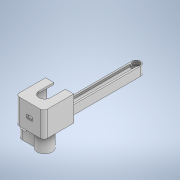
# Autodesk Inventor part: motor-rack
Saved by Autodesk Inventor 2021 (Build 250183000, 183)
## iProperties
Created: 2024-04-10
Part Number: motor-rack
Material: Generic
Document SubType Name: Modeling
Designer: 22hamfri
Density: 1 g/cm^3
Appearance: Default
Author: 22hamfri
Autodesk Inventor part; units mm, degrees
ref_plane "YZ Plane" through (0, 0, 0) normal (1, 0, 0) x (0, 1, 0)
ref_plane "XZ Plane" through (0, 0, 0) normal (0, 1, 0) x (-1, 0, 0)
ref_plane "XY Plane" through (0, 0, 0) normal (0, 0, 1) x (1, 0, 0)
sketch "Sketch1" plane through (0, 0, 0) normal (0, 1, 0) x (-1, 0, 0)
  circle A0 centre (0, -95.64) radius 2.575
  circle A1 centre (0, -95.64) radius 3.1
  circle A2 centre (0, -95.64) radius 3.8
  circle A3 centre (-15.94, 0) radius 2.575
  circle A4 centre (-15.94, 0) radius 3.1
  circle A5 centre (-15.94, 0) radius 3.8
  circle A6 centre (0, 0) radius 3.8
  line L0 (0, 0) -> (0, -95.64)
  line L1 (0, 0) -> (-15.94, 0)
  line L2 (3.8, 0) -> (3.8, -95.64)
  line L3 (-3.8, 0) -> (-3.8, -95.64)
  line L4 (0, 3.8) -> (-15.94, 3.8)
  line L5 (0, -3.8) -> (-15.94, -3.8)
  arc A7 (-3.8, -4.8) -> (-4.8, -3.8) centre (-4.8, -4.8) ccw
  line L6 (-12.9151, 2.3) -> (0, 2.3)
  line L7 (2.3, 0) -> (2.3, -92.6151)
  circle A8 centre (0, 0) radius 2.3
  arc A9 (-2.3, -4.8) -> (-4.8, -2.3) centre (-4.8, -4.8) ccw
  line L8 (-4.8, -2.3) -> (-12.9151, -2.3)
  line L9 (-2.3, -4.8) -> (-2.3, -92.6151)
  dimension "d0" = 0.7
  dimension "d1" = 6.2
  dimension "d2" = 5.15
  dimension "d3" = 0.7
  dimension "d4" = 5.15
  dimension "d5" = 6.2
  dimension "d6" = 7.6
  dimension "d7" = 95.64
  dimension "d8" = 15.94
  dimension "d9" = 1
  dimension "d10" = 1.5
  dimension "d11" = 1.5
  constraints: 20 end point, 18 point on circle, 12 tangent, 10 centre point, 4 point on line, 3 horizontal, 2 vertical, 1 coincident, 1 parallel
  measures "d0" radial gap between concentric circles of A1 A2
  measures "d1" diameter of A1
  measures "d2" diameter of A0
  measures "d3" radial gap between concentric circles of A4 A5
  measures "d4" diameter of A3
  measures "d5" diameter of A4
  measures "d6" diameter of A6
  measures "d7" distance of L0.start L0.end
  measures "d8" distance of L0.start L1.end
  measures "d9" radius of A7
  measures "d10" radial gap between concentric circles of A6 A8
  measures "d11" radial gap between concentric circles of A7 A9
extrude "Extrusion1" add sketch "Sketch1" against normal mid plane 7.76 contours A2 | A2 L7 A6 L2 | L3 L5 A9 L9 A2 | A6 L7 A8 L6 | A7 L5 L3 | A6 L6 A5 L4 | L5 A5 L8 A9 L3 | L3 A9 L5 | A5
extrude "Extrusion2" add sketch "Sketch1" against normal mid plane 6.16 contours A1 | A4
extrude "Extrusion3" add sketch "Sketch1" against normal mid plane 4 contours A2 L0 A6 L7 | A2 L9 A9 L5 L0 | A6 L0 A8 L7 | L5 A9 L3 A6 | A6 L1 A8 L0 | A8 L0 L1 | L6 A8 L1 A6 | A6 L1 A5 L6 | L3 A9 L8 A5 L1 | A8 L1 L0
sketch "Sketch2" plane through (0, 3.88, 0) normal (0, 1, 0) x (1, 0, 0)
  arc A0 (3.8, 4.8) -> (4.8, 3.8) centre (4.8, 4.8) ccw projected
  line L0 (3.8, 4.8) -> (3.8, 95.64) projected
  arc A1 (3.8, 95.64) -> (-3.8, 95.64) centre (0, 95.64) ccw projected
  line L1 (-3.8, 95.64) -> (-3.8, 0) projected
  arc A2 (-3.8, 0) -> (0, -3.8) centre (0, 0) ccw projected
  line L2 (0, -3.8) -> (15.94, -3.8) projected
  arc A3 (15.94, -3.8) -> (15.94, 3.8) centre (15.94, 0) ccw projected
  line L3 (15.94, 3.8) -> (4.8, 3.8) projected
  circle A4 centre (0, 95.64) radius 3.1 projected
  circle A5 centre (15.94, 0) radius 3.1 projected
  arc A6 (-2.3, 92.6151) -> (2.3, 92.6151) centre (0, 95.64) ccw projected
  line L4 (2.3, 92.6151) -> (2.3, 4.8) projected
  arc A7 (2.3, 4.8) -> (4.8, 2.3) centre (4.8, 4.8) ccw projected
  line L5 (4.8, 2.3) -> (12.9151, 2.3) projected
  arc A8 (12.9151, 2.3) -> (12.9151, -2.3) centre (15.94, 0) ccw projected
  line L6 (12.9151, -2.3) -> (0, -2.3) projected
  arc A9 (-2.3, 0) -> (0, -2.3) centre (0, 0) ccw projected
  line L7 (-2.3, 0) -> (-2.3, 92.6151) projected
  circle A10 centre (15.94, 0) radius 6.5
  dimension "d40" = 13
  constraints: 1 centre point
  measures "d40" diameter of A10
extrude "Extrusion4" cut sketch "Sketch2" against normal blind 5 contours A10 L2 A3 L3 | L3 A3 L2 A10 L6 A8 L5 | L5 A8 L6 A10 | A5
sketch "Sketch3" plane through (0, -1.12, 0) normal (0, 1, 0) x (1, 0, 0)
  arc A0 (10.6665, 3.8) -> (9.8605, 2.3) centre (15.94, 0) ccw projected
  arc A1 (9.8605, 2.3) -> (9.8605, -2.3) centre (15.94, 0) ccw projected
  arc A2 (9.8605, -2.3) -> (10.6665, -3.8) centre (15.94, 0) ccw projected
  arc A3 (10.6665, 3.8) -> (10.6665, -3.8) centre (15.94, 0) ccw projected
  circle A4 centre (15.94, 0) radius 6.5
  arc A5 (10.6665, 3.8) -> (10.6665, -3.8) centre (15.94, 0) ccw projected
  circle A6 centre (15.94, 0) radius 5
  line L0 (10.6665, 3.8) -> (15.94, 3.8) projected
  arc A7 (10.6665, 3.8) -> (10.6665, -3.8) centre (15.94, 0) ccw projected
  line L1 (15.94, -3.8) -> (10.6665, -3.8) projected
  arc A8 (15.94, -3.8) -> (15.94, 3.8) centre (15.94, 0) ccw projected
  circle A9 centre (15.94, 0) radius 2.575 projected
  line L2 (20.94, 0) -> (20.94, 4.1533)
  line L3 (10.94, 0) -> (10.94, 4.1533)
  point P0 (0, 0)
  point P1 (10.6665, -3.8)
  point P2 (10.6665, 3.8)
  point P3 (9.8605, 2.3)
  point P4 (9.8605, -2.3)
  dimension "d20" = 1.5
  constraints: 4 end point, 4 point on circle, 3 tangent, 2 centre point, 2 vertical, 1 coincident
  measures "d20" radial gap between concentric circles of A4 A6
extrude "Extrusion5" add sketch "Sketch3" against normal up to surface (2.76 mm away) contours A4 L3 L0 | A4 L2 A6 L0 L3 | A4 L1 A6 L2 | A6 L1 A8 L0 picked at (14.0877, -4.0119)
extrude "Extrusion6" add sketch "Sketch3" along normal blind 17 contours L0 L3 A6 L1 A2 A1 A0 | A4 L3 L0 | A4 L1 A6 L2
sketch "Sketch4" plane through (0, 15.88, 0) normal (0, 1, 0) x (1, 0, 0)
  arc A0 (10.94, 0) -> (20.94, 0) centre (15.94, 0) ccw projected
  line L0 (4.69, 12) -> (27.19, 12)
  line L1 (27.19, 12) -> (27.19, -10)
  line L2 (25.19, -12) -> (6.69, -12)
  line L3 (4.69, -10) -> (4.69, 12)
  line L4 (4.69, 12) -> (27.19, -12) construction
  line L5 (27.19, 12) -> (4.69, -12) construction
  arc A1 (4.69, -10) -> (6.69, -12) centre (6.69, -10) ccw
  arc A2 (25.19, -12) -> (27.19, -10) centre (25.19, -10) ccw
  line L6 (4.69, 12) -> (4.69, 13)
  line L7 (4.69, 13) -> (27.19, 13)
  line L8 (27.19, 13) -> (27.19, 12)
  line L9 (3.69, 13) -> (3.69, -10)
  arc A3 (3.69, -10) -> (6.69, -13) centre (6.69, -10) ccw
  line L10 (6.69, -13) -> (25.19, -13)
  arc A4 (25.19, -13) -> (28.19, -10) centre (25.19, -10) ccw
  line L11 (28.19, -10) -> (28.19, 13)
  line L12 (28.19, 13) -> (27.19, 13)
  line L13 (3.69, 13) -> (4.69, 13)
  line L14 (10.94, 0) -> (10.94, 4.1533) projected
  arc A5 (10.94, 4.1533) -> (20.94, 4.1533) centre (15.94, 0) ccw projected
  line L15 (20.94, 4.1533) -> (20.94, 0) projected
  line L16 (20.94, 4.1533) -> (20.94, 0) projected
  line L17 (20.94, 4.1533) -> (20.94, 13)
  line L18 (10.94, 0) -> (10.94, 4.1533) projected
  line L19 (10.94, 4.1533) -> (10.94, 13)
  point P0 (0, 0)
  point P1 (15.94, 0)
  dimension "d26" = 22.5
  dimension "d27" = 12
  dimension "d28" = 2
  dimension "d29" = 2
  dimension "d30" = 25
  dimension "d31" = 1
  constraints: 32 end point, 8 point on circle, 8 point on line, 4 centre point, 4 perpendicular, 4 tangent, 3 parallel, 2 horizontal, 2 midpoint, 1 coincident, 1 vertical, 4 other
  measures "d26" distance between parallel lines of L1 L3
  measures "d27" distance from line of L2 A0.centre
  measures "d28" radius of A1
  measures "d29" radius of A2
  measures "d30" distance between parallel lines of L7 L2
  measures "d31" distance between parallel lines of L1 L11
extrude "Extrusion7" add sketch "Sketch4" against normal blind 1.5 contours A5 L17 L0 L1 A2 L2 A1 L3 L19 | L0 L6 L7 L19 | L17 L7 L8 L0 | L3 A1 L2 A2 L1 L8 L12 L11 A4 L10 A3 L9 L13 L6
extrude "Extrusion8" add sketch "Sketch4" along normal blind 19 contours L3 A1 L2 A2 L1 L8 L12 L11 A4 L10 A3 L9 L13 L6
sketch "Sketch5" plane through (0, 34.88, 0) normal (0, 1, 0) x (1, 0, 0)
  line L0 (3.69, 13) -> (3.69, -10) projected
  arc A0 (3.69, -10) -> (6.69, -13) centre (6.69, -10) ccw projected
  line L1 (6.69, -13) -> (25.19, -13) projected
  arc A1 (25.19, -13) -> (28.19, -10) centre (25.19, -10) ccw projected
  line L2 (28.19, -10) -> (28.19, 13) projected
  line L3 (28.19, 13) -> (27.19, 13) projected
  line L4 (27.19, 13) -> (27.19, -10) projected
  arc A2 (25.19, -12) -> (27.19, -10) centre (25.19, -10) ccw projected
  line L5 (25.19, -12) -> (6.69, -12) projected
  arc A3 (4.69, -10) -> (6.69, -12) centre (6.69, -10) ccw projected
  line L6 (4.69, -10) -> (4.69, 13) projected
  line L7 (4.69, 13) -> (3.69, 13) projected
  line L8 (27.19, -10) -> (27.19, 13) projected
  line L9 (27.19, 13) -> (20.94, 13) projected
  line L10 (20.94, 13) -> (20.94, 0) projected
  arc A4 (10.94, 0) -> (20.94, 0) centre (15.94, 0) ccw projected
  line L11 (10.94, 0) -> (10.94, 13) projected
  line L12 (10.94, 13) -> (4.69, 13) projected
  line L13 (4.69, 13) -> (4.69, -10) projected
  arc A5 (4.69, -10) -> (6.69, -12) centre (6.69, -10) ccw projected
  line L14 (6.69, -12) -> (25.19, -12) projected
  arc A6 (25.19, -12) -> (27.19, -10) centre (25.19, -10) ccw projected
extrude "Extrusion9" add sketch "Sketch5" along normal blind 1.5
sketch "Sketch6" plane through (0, 3.88, 0) normal (0, 1, 0) x (1, 0, 0)
  arc A0 (10.6665, 3.8) -> (9.8605, 2.3) centre (15.94, 0) ccw projected
  line L0 (10.6665, 3.8) -> (4.8, 3.8) projected
  arc A1 (3.8, 4.8) -> (4.8, 3.8) centre (4.8, 4.8) ccw projected
  line L1 (3.8, 4.8) -> (3.8, 95.64) projected
  arc A2 (3.8, 95.64) -> (-3.8, 95.64) centre (0, 95.64) ccw projected
  line L2 (-3.8, 95.64) -> (-3.8, 0) projected
  arc A3 (-3.8, 0) -> (0, -3.8) centre (0, 0) ccw projected
  line L3 (0, -3.8) -> (10.6665, -3.8) projected
  arc A4 (9.8605, -2.3) -> (10.6665, -3.8) centre (15.94, 0) ccw projected
  line L4 (9.8605, -2.3) -> (0, -2.3) projected
  arc A5 (-2.3, 0) -> (0, -2.3) centre (0, 0) ccw projected
  line L5 (-2.3, 0) -> (-2.3, 92.6151) projected
  arc A6 (-2.3, 92.6151) -> (2.3, 92.6151) centre (0, 95.64) ccw projected
  line L6 (2.3, 92.6151) -> (2.3, 4.8) projected
  arc A7 (2.3, 4.8) -> (4.8, 2.3) centre (4.8, 4.8) ccw projected
  line L7 (4.8, 2.3) -> (9.8605, 2.3) projected
  circle A8 centre (0, 95.64) radius 3.1 projected
  arc A9 (10.94, 4.1533) -> (20.94, 4.1533) centre (15.94, 0) ccw projected
  line L8 (20.94, 13) -> (28.19, 13) projected
  line L9 (28.19, 13) -> (28.19, -10) projected
  arc A10 (25.19, -13) -> (28.19, -10) centre (25.19, -10) ccw projected
  line L10 (25.19, -13) -> (6.69, -13) projected
  arc A11 (3.69, -10) -> (6.69, -13) centre (6.69, -10) ccw projected
  line L11 (3.69, -10) -> (3.69, 13) projected
  line L12 (10.6665, 3.8) -> (4.8, 3.8) projected
  line L13 (4.8, 3.8) -> (3.69, 3.8)
  line L14 (10.94, 13) -> (10.94, 4.1533) projected
  line L15 (20.94, 4.1533) -> (20.94, 13) projected
  line L16 (3.69, 13) -> (10.94, 13) projected
  point P0 (3.69, -2.3)
  point P1 (3.69, -3.8)
  point P2 (3.69, 2.5599)
  constraints: 2 end point, 1 perpendicular, 1 point on line
extrude "Extrusion10" add sketch "Sketch6" along normal up to surface (10.5 mm away) contours A0 L7 A7 L11 L13 L0 | A4 L3 L11 L4
sketch "Sketch7" plane through (25.19, 15.88, 12) normal (0, 0, -1) x (-1, 0, 0)
  line L0 (18.5, 0) -> (0, 0) projected
  line L1 (18.5, 0) -> (18.5, 19) projected
  line L2 (0, 19) -> (18.5, 19) projected
  line L3 (0, 0) -> (0, 19) projected
  line L4 (6.75, 8) -> (11.75, 8)
  line L5 (11.75, 8) -> (11.75, 11)
  line L6 (11.75, 11) -> (6.75, 11)
  line L7 (6.75, 11) -> (6.75, 8)
  line L8 (6.75, 8) -> (11.75, 11) construction
  line L9 (11.75, 8) -> (6.75, 11) construction
  line L10 (9.25, 9.5) -> (18.5, 9.5)
  line L11 (18.5, -1.5) -> (18.5, 20.5) projected
  line L12 (9.25, 9.5) -> (0, 9.5)
  line L13 (0, -1.5) -> (0, 20.5) projected
  line L14 (9.25, 9.5) -> (9.25, 19)
  line L15 (0, 19) -> (18.5, 19) projected
  line L16 (9.25, 9.5) -> (9.25, 0)
  line L17 (18.5, 0) -> (0, 0) projected
  point P0 (25.19, -15.88)
  dimension "d41" = 5
  dimension "d42" = 3
  constraints: 20 end point, 6 midpoint, 2 collinear, 2 parallel, 1 horizontal, 1 perpendicular
  measures "d41" distance of L4.start L4.end
  measures "d42" distance of L4.end L5.end
extrude "Extrusion11" cut sketch "Sketch7" against normal up to surface (1 mm away) contours L16 L10 L5 L4 | L4 L7 L12 L16 | L10 L14 L6 L5 | L12 L7 L6 L14
body "Solid1"
